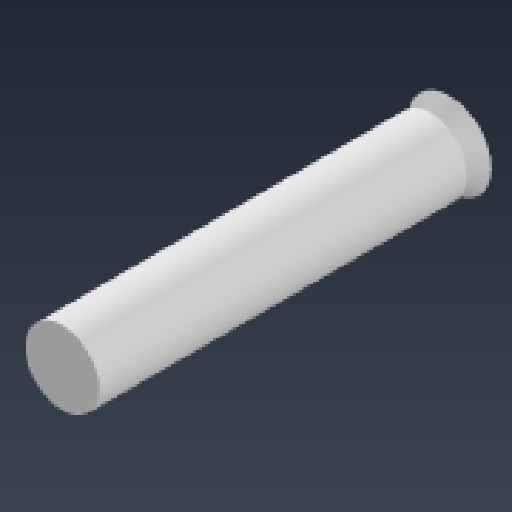
# Autodesk Inventor part: m3 spacer bolt combo
Saved by Autodesk Inventor 2024.3 (Build 283343000, 343)
## iProperties
Created: 2024-10-06
Part Number: m3 spacer bolt combo
Material: Generic
Document SubType Name: Modeling
Designer: MFil
Density: 1 g/cm^3
Appearance: Default
Author: MFil
Autodesk Inventor part; units mm, degrees
ref_plane "YZ Plane" through (0, 0, 0) normal (1, 0, 0) x (0, 1, 0)
ref_plane "XZ Plane" through (0, 0, 0) normal (0, 1, 0) x (-1, 0, 0)
ref_plane "XY Plane" through (0, 0, 0) normal (0, 0, 1) x (1, 0, 0)
sketch "Sketch1" plane through (0, 0, 0) normal (0, 1, 0) x (-1, 0, 0)
  line L0 (0, 0) -> (2.5, 0)
  line L1 (2.5, 0) -> (2.5, -25)
  line L2 (2.5, -25) -> (0, -25)
  line L3 (0, -25) -> (0, 0)
  line L4 (0, -25) -> (2.775, -25)
  line L5 (0, -26.3) -> (2.85, -26.3)
  line L6 (2.85, -26.3) -> (1.55, -25)
  line L7 (2.85, -26.3) -> (4.6885, -26.3) construction
  line L8 (0, -26.3) -> (0, -25)
  dimension "d1" = 25
  dimension "d2" = 2.775
  dimension "d20" = 2.85
  dimension "d21" = 1.3
  dimension "d22" = 135
  constraints: 18 end point, 4 horizontal, 2 parallel, 1 equal length, 1 perpendicular, 1 point on line, 1 vertical
  measures "d1" distance of L0.end L1.end
  measures "d2" distance of L2.end L4.end
  measures "d20" distance of L5.start L5.end
  measures "d21" distance between parallel lines of L5 L2
  measures "d22" angle of L7 L6
revolve "Revolution1" add sketch "Sketch1" angle 360 about axis through (0, 0, -25) along (0, 0, 1)
sketch "Sketch4" plane through (0, 0, -26.3) normal (0, 0, -1) x (-1, 0, 0)
  circle A0 centre (0, 0) radius 1.55 projected
  line L0 (0, 1.1547) -> (1, 0.5774)
  line L1 (1, 0.5774) -> (1, -0.5774)
  line L2 (1, -0.5774) -> (0, -1.1547)
  line L3 (0, -1.1547) -> (-1, -0.5774)
  line L4 (-1, -0.5774) -> (-1, 0.5774)
  line L5 (-1, 0.5774) -> (0, 1.1547)
  dimension "d23" = 2
  constraints: 12 end point, 1 coincident, 13 other
  measures "d23" distance between parallel lines of L1 L4
extrude "Extrusion2" cut sketch "Sketch4" against normal blind 1.2 contours L0 L1 L2 L3 L4 L5
body "Solid1"
